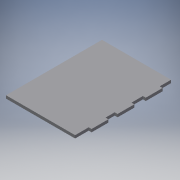
# Autodesk Inventor part: back
Saved by Autodesk Inventor 2016 (Build 200138000, 138)
## iProperties
Created: 2016-05-17
Part Number: back
Material: Generic
Document SubType Name: Modeling
Designer: Lillahunden
Density: 1 g/cm^3
Appearance: Default
Author: Lillahunden
Autodesk Inventor part; units mm, degrees
ref_plane "YZ Plane" through (0, 0, 0) normal (1, 0, 0) x (0, 1, 0)
ref_plane "XZ Plane" through (0, 0, 0) normal (0, 1, 0) x (-1, 0, 0)
ref_plane "XY Plane" through (0, 0, 0) normal (0, 0, 1) x (1, 0, 0)
sketch "Sketch1" plane through (0, 0, 0) normal (0, 0, 1) x (1, 0, 0)
  line L0 (0, -63.3717) -> (0, -35) projected
  line L1 (0, -35) -> (-6, -35) projected
  line L2 (-6, -63.3717) -> (-6, -35) projected
  line L3 (0, -63.3717) -> (-6, -63.3717) projected
  line L4 (0, -35) -> (0, 0) projected
  line L5 (0, 0) -> (-6, 0) projected
  line L6 (-6, -35) -> (-6, 0) projected
  line L7 (0, -35) -> (-6, -35) projected
  line L8 (-6, 0) -> (-6, 19.1283) projected
  line L9 (0, 19.1283) -> (0, 54.1283) projected
  line L10 (0, 54.1283) -> (-6, 54.1283) projected
  line L11 (-6, 19.1283) -> (-6, 54.1283) projected
  line L12 (0, 19.1283) -> (-6, 19.1283) projected
  line L13 (0, 0) -> (0, 19.1283) projected
  line L14 (0, 19.1283) -> (-6, 19.1283) projected
  line L15 (-6, 0) -> (-6, 19.1283) projected
  line L16 (0, 0) -> (-6, 0) projected
  line L17 (0, 54.1283) -> (0, 77.8783) projected
  line L18 (0, 77.8783) -> (-6, 77.8783) projected
  line L19 (-6, 54.1283) -> (-6, 77.8783) projected
  line L20 (0, 54.1283) -> (-6, 54.1283) projected
  line L21 (0, 77.8783) -> (0, 112.8783) projected
  line L22 (0, 112.8783) -> (-6, 112.8783) projected
  line L23 (-6, 77.8783) -> (-6, 112.8783) projected
  line L24 (0, 77.8783) -> (-6, 77.8783) projected
  line L25 (0, 112.8783) -> (0, 136.6283) projected
  line L26 (0, 136.6283) -> (-6, 136.6283) projected
  line L27 (-6, 112.8783) -> (-6, 136.6283) projected
  line L28 (0, 112.8783) -> (-6, 112.8783) projected
  line L29 (0, -63.3717) -> (-150, -63.3717)
  line L30 (-150, -63.3717) -> (-150, 136.6283)
  line L31 (-150, 136.6283) -> (0, 136.6283)
  line L32 (0, 136.6283) -> (0, -63.3717)
  dimension "d0" = 150
  constraints: 8 end point, 2 parallel, 1 horizontal, 1 perpendicular
  measures "d0" distance of L30.end L31.end
extrude "Extrusion1" add sketch "Sketch1" along normal blind 6 contours L1 L6 L5 L4 | L29 L30 L31 L27 L23 L19 L11 L8 L6 L2 | L12 L11 L10 L9 | L18 L23 L22 L21
body "Solid1"
